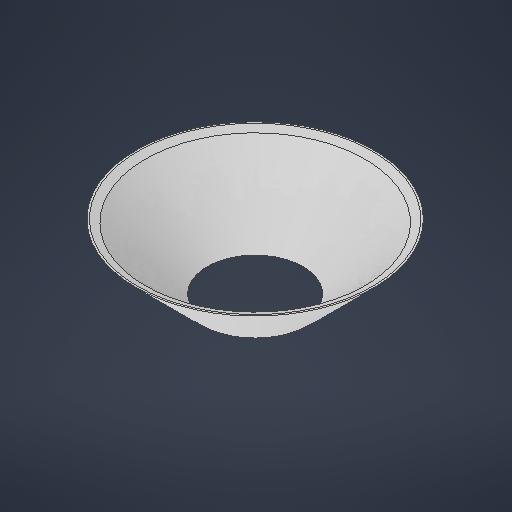
# Autodesk Inventor part: basket
Saved by Autodesk Inventor 2026.2 (Build 302298010, 298A)
## iProperties
Created: 2026-03-21
Part Number: basket
Material: Generic
Document SubType Name: Modeling
Designer: Amir
Density: 1 g/cm^3
Appearance: Default
Author: Amir
## iProperties of the stored document basket_3DPrint.ipt
Created: 2026-04-17
Part Number: basket_3DPrint
Material: Generic
Document SubType Name: Modeling
Designer: lenovo
Density: 1 g/cm^3
Appearance: Default
Author: lenovo
Autodesk Inventor part; units mm, degrees
ref_plane "YZ Plane" through (0, 0, 0) normal (1, 0, 0) x (0, 1, 0)
ref_plane "XZ Plane" through (0, 0, 0) normal (0, 1, 0) x (-1, 0, 0)
ref_plane "XY Plane" through (0, 0, 0) normal (0, 0, 1) x (1, 0, 0)
sketch "Sketch3" plane through (0, 0, 0) normal (0, 0, 1) x (1, 0, 0)
  line L0 (-4.8838, 52) -> (25.1162, 22)
  line L1 (-4.8838, 52) -> (-4.8838, 54.8284)
  line L2 (-10.9325, 0) -> (57.9097, 0)
  line L3 (-4.8838, 54.8284) -> (25.1162, 24.8284)
  line L4 (-4.8838, 52) -> (-4.8838, 37.7002) construction
  line L5 (25.1162, 24.8284) -> (25.1162, 22)
  point P0 (0, 0)
  point P1 (23.4886, 0)
  point P2 (25.1162, 23.4142)
  point P3 (-4.8838, 53.4142)
  dimension "d32" = 2
  dimension "d39" = 22
  dimension "d44" = 45
  dimension "d45" = 30
  constraints: 12 end point, 3 midpoint, 3 vertical, 1 horizontal, 1 horizontal alignment, 1 parallel
  measures "d32" distance between parallel lines of L0 L3
  measures "d39" distance from line of L0.end L2
  measures "d44" angle of L0 L4
  measures "d45" horizontal distance of point (25.116, 23.414) point (-4.884, 53.414)
revolve "Revolution1" add sketch "Sketch3" angle 360 about axis through (-10.9325, 0, 0) along (1, 0, 0)
chamfer "Chamfer1" distance 2 angle 45 1 edges at (-4.8838, -52, 0)
body "Solid2"
